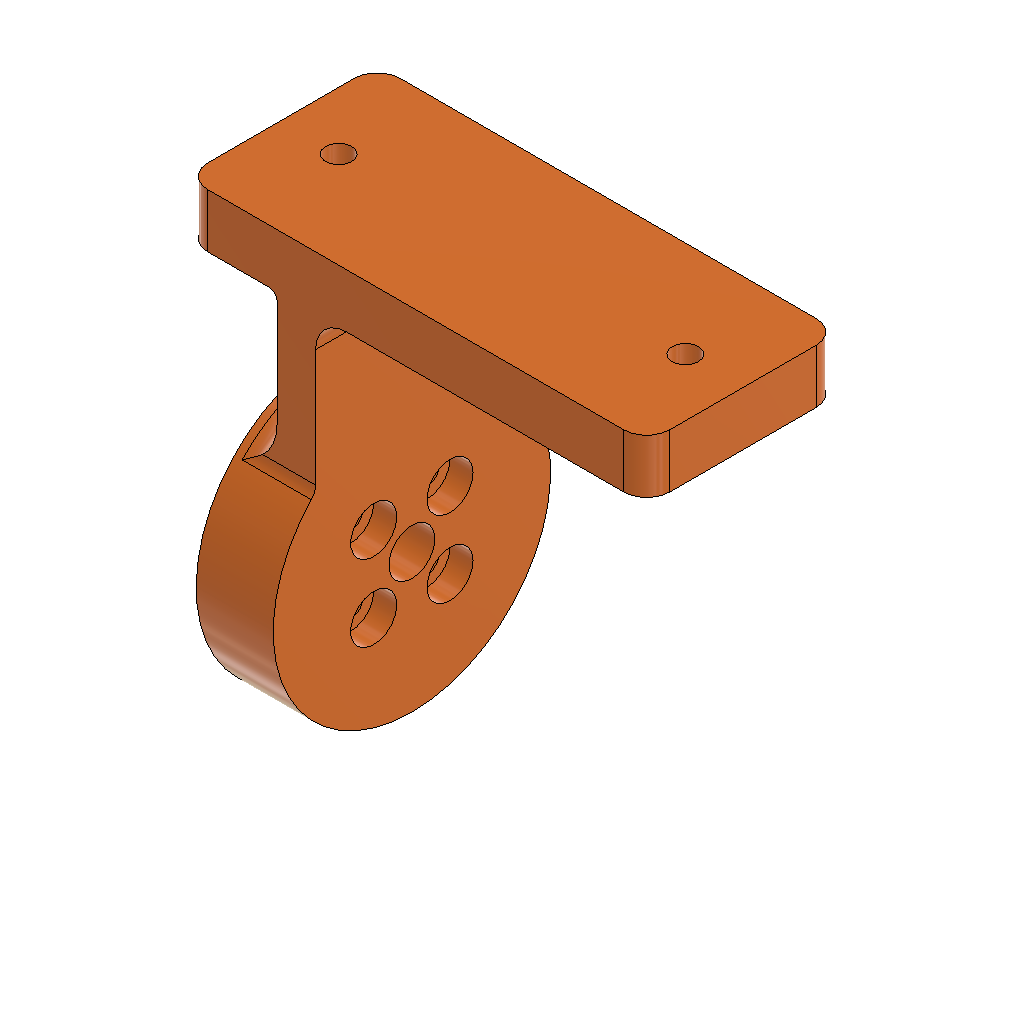
head_cam_mount_d435i (Autodesk Fusion 360 design; units mm, degrees)
part number: 2026-10-04-09-41-25-505
Autodesk Fusion 360 part; units mm, degrees
ref_plane "作業平面2" through (-13, 0, 0) normal (1, 0, 0) x (0, 1, 0)
sketch "スケッチ5" plane through (-13, 0, 0) normal (1, 0, 0) x (0, 0, -1)
  circle A0 centre (0, 0) radius 18
  circle A1 centre (0, 0) radius 9.5
  dimension "d120" = 36
  dimension "d121" = 19
  measures "d120" diameter of A0
  measures "d121" diameter of A1
extrude "disc" add sketch "スケッチ5" against normal blind 10 contours A0 | A1 makes body 1
extrude "boss" add sketch "スケッチ5" against normal blind 4.8 from surface at -10 contours A1 bodies 1
sketch "スケッチ6" plane through (-13, 0, 0) normal (1, 0, 0) x (0, 0, -1)
  line L0 (4.9497, -4.9497) -> (-4.9497, 4.9497) construction
  line L1 (-4.9497, -4.9497) -> (4.9497, 4.9497) construction
  dimension "d127" = 9.8995
  dimension "d128" = 9.8995
  dimension "d129" = 9.8995
  dimension "d130" = 9.8995
  constraint midpoint origin L0
  constraint midpoint origin L1
  measures "d127" horizontal distance of L0.start L0.end
  measures "d128" vertical distance of L0.start L0.end
  measures "d129" horizontal distance of L1.start L1.end
  measures "d130" vertical distance of L1.start L1.end
hole "horn_holes" at (-13, -4.9497, -4.9497) at (-13, 4.9497, 4.9497) at (-13, -4.9497, 4.9497) at (-13, 4.9497, -4.9497) direction (-1, 0, 0) diameter 3.2 end through all counterbore diameter 6 counterbore depth 3 bodies 1
hole "center_hole" at (-13, 0, 0) direction (-1, 0, 0) diameter 6 end through all bodies 1
ref_plane "作業平面1" through (0, 0, 33) normal (0, 0, 1) x (1, 0, 0)
sketch "スケッチ1" plane through (0, 0, 33) normal (0, 0, 1) x (1, 0, 0)
  line L0 (-30, -12.5) -> (30, -12.5)
  line L1 (30, -12.5) -> (30, 12.5)
  line L2 (30, 12.5) -> (-30, 12.5)
  line L3 (-30, 12.5) -> (-30, -12.5)
  line L4 (-22.5, 0) -> (22.5, 0) construction
  circle A0 centre (-22.5, 0) radius 1.7
  circle A1 centre (22.5, 0) radius 1.7
  dimension "d22" = 12.5
  dimension "d23" = 30
  dimension "d24" = 12.5
  dimension "d25" = 30
  dimension "d26" = 45
  dimension "d27" = 3.4
  dimension "d28" = 3.4
  constraint horizontal L4
  constraint midpoint origin L4
  constraint horizontal L0
  constraint vertical L1
  constraint horizontal L2
  constraint vertical L3
  measures "d22" vertical distance of origin L0.start
  measures "d23" horizontal distance of origin L0.end
  measures "d24" vertical distance of origin L1.end
  measures "d25" horizontal distance of origin L2.end
  measures "d26" horizontal distance of L4.start L4.end
  measures "d27" diameter of A0
  measures "d28" diameter of A1
extrude "camera_plate" add sketch "スケッチ1" along normal blind 7 separate body makes body 2
fillet "plate_corner_fillet" radius 3 4 edges at (-30, 12.5, 36.5) (30, 12.5, 36.5) (30, -12.5, 36.5) (-30, -12.5, 36.5) on bodies 2
sketch "スケッチ4" plane through (0, 0, 0) normal (0, 1, 0) x (1, 0, 0)
  line L0 (-18, -12) -> (-13, -12)
  line L1 (-13, -12) -> (-13, -33)
  line L2 (-13, -33) -> (-18, -33)
  line L3 (-18, -33) -> (-18, -12)
  dimension "d75" = 13
  dimension "d76" = 5
  dimension "d77" = 12
  dimension "d78" = 33
  constraint horizontal L0
  constraint vertical L1
  constraint horizontal L2
  constraint vertical L3
  measures "d75" horizontal distance of origin L0.end
  measures "d76" horizontal distance of L0.end L2.end
  measures "d77" vertical distance of origin L0.start
  measures "d78" vertical distance of origin L1.end
extrude "web" add sketch "スケッチ4" along normal mid plane 25 separate body makes body 3
combine "join_disc_plate_web" operation add target body 1 tool bodies 2 3
fillet "junction_fillets" radius 4 1 edges at (-13, 0, 33) on bodies 1
fillet "junction_fillets" radius 1 1 edges at (-18, 0, 33) on bodies 1
fillet "junction_fillets" radius 2 2 edges at (-15.5, 12.5, 12.9518) (-15.5, -12.5, 12.9518) on bodies 1
fillet "rim_web_fillet_lane_side" radius 4 1 edges at (-18, 0, 18) on bodies 1
equation "d20 = forward_offset - plate_thickness"
equation "d22 = plate_height / 2"
equation "d23 = plate_width / 2"
equation "d24 = plate_height / 2"
equation "d25 = plate_width / 2"
equation "d26 = hole_spacing"
equation "d27 = hole_dia"
equation "d28 = hole_dia"
equation "d29 = plate_thickness"
equation "d32 = plate_corner_r"
equation "d75 = disc_offset"
equation "d76 = web_thickness"
equation "d77 = web_back_z"
equation "d78 = forward_offset - plate_thickness"
equation "d79 = plate_height"
equation "d118 = -disc_offset"
equation "d120 = disc_dia"
equation "d121 = boss_dia"
equation "d122 = -( disc_thickness )"
equation "d124 = -disc_thickness"
equation "d125 = -( boss_height )"
equation "d127 = horn_pcd / sqrt(2)"
equation "d128 = horn_pcd / sqrt(2)"
equation "d129 = horn_pcd / sqrt(2)"
equation "d130 = horn_pcd / sqrt(2)"
equation "d131 = horn_hole_dia"
equation "d133 = horn_cbore_depth"
equation "d134 = horn_cbore_dia"
equation "d135 = center_hole_dia"
equation "d138 = fillet_r"
equation "d140 = fillet_lane_r"
equation "d142 = fillet_r / 2"
equation "d144 = rim_fillet_r"
equation "forward_offset = 40 mm" comment "Camera back face distance in front of the tilt axis"
equation "plate_thickness = 7 mm" comment "Camera plate thickness (M3x10, no counterbore -> 3 mm engagement)"
equation "plate_width = 60 mm" comment "Camera plate width (X)"
equation "plate_height = 25 mm" comment "Camera plate height (Y), equals camera height"
equation "plate_corner_r = 3 mm" comment "Camera plate corner radius"
equation "hole_dia = 3.4 mm" comment "Camera screw clearance hole (M3 + 0.4)"
equation "hole_spacing = 45 mm" comment "D435i rear M3 hole spacing"
equation "web_back_z = 12 mm" comment "Web rear end Z (web joins the disc only at its rim; keeps the horn screws reachable along +X)"
equation "fillet_r = 4 mm" comment "Fillet radius at the arm-plate junction"
equation "web_thickness = 5 mm" comment "Vertical web thickness (X)"
equation "fillet_lane_r = 1 mm" comment "Fillet between the web -X face and the plate back face (screw lane side)"
equation "disc_dia = 36 mm" comment "Horn disc diameter (HeadCamMount)"
equation "disc_thickness = 10 mm" comment "Horn disc thickness (X)"
equation "disc_offset = 13 mm" comment "Pan axis to the disc +X face (horn screw side); disc spans x = -(disc_offset+disc_thickness) .. -disc_offset"
equation "boss_dia = 19 mm" comment "Horn-side boss diameter (passes through the AXK2035 bore)"
equation "boss_height = 4.8 mm" comment "Horn-side boss height (-X)"
equation "horn_hole_dia = 3.2 mm" comment "Horn screw clearance hole"
equation "horn_pcd = 14 mm" comment "Horn screw PCD (9.9 mm square)"
equation "horn_cbore_dia = 6 mm" comment "Horn screw counterbore diameter (+X face)"
equation "horn_cbore_depth = 3 mm" comment "Horn screw counterbore depth"
equation "center_hole_dia = 6 mm" comment "Center through hole (horn center screw access)"
equation "rim_fillet_r = 4 mm" comment "Fillet between the disc rim and the web -X face (screw lane side)"
named bodies: "plate_tmp", "web_tmp", "head_cam_mount_d435i"
